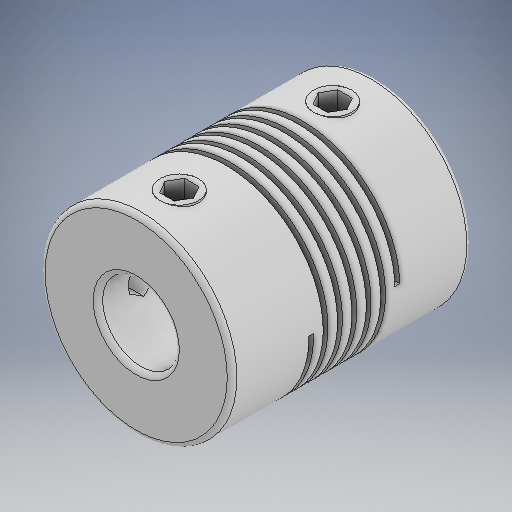
# Autodesk Inventor part: shaft_coupler 5mm_to_8mm
Saved by Autodesk Inventor 2025.2 (Build 292293000, 293)
## iProperties
Created: 2025-04-06
Part Number: shaft_coupler 5mm_to_8mm
Material: Generic
Document SubType Name: Modeling
Designer: Tiago
Density: 1 g/cm^3
Appearance: Default
Author: Tiago
Autodesk Inventor part; units mm, degrees
sketch "Sketch1" plane through (0, 0, 0) normal (0, 0, 1) x (1, 0, 0)
  circle A0 centre (0, 0) radius 10
  circle A1 centre (0, 0) radius 2.5
  dimension "D" = 20
  dimension "di1" = 5
  constraints: 2 centre point, 2 coincident
  measures "D" diameter of A0
  measures "di1" diameter of A1
ref_plane "Work Plane1" through (0, 0, 25) normal (0, 0, 1) x (1, 0, 0)
sketch "Sketch2" plane through (0, 0, 25) normal (0, 0, 1) x (1, 0, 0)
  circle A0 centre (0, 0) radius 4
  circle A1 centre (0, 0) radius 10
  dimension "di2" = 8
  dimension "d4" = 20
  constraints: 2 centre point, 2 coincident
  measures "di2" diameter of A0
  measures "d4" diameter of A1
extrude "Extrusion1" add sketch "Sketch2" against normal up to surface (25 mm away)
extrude "Extrusion2" add sketch "Sketch1" along normal blind 10
ref_plane "Work Plane2" through (-10, 0, 0) normal (1, 0, 0) x (0, 1, 0)
sketch "Sketch3" plane through (-10, 0, 0) normal (1, 0, 0) x (0, 1, 0)
  line L0 (0, 0) -> (0, 25) construction
  line L1 (-4, 25) -> (4, 25) construction
  line L2 (0, 20.5) -> (0, 4.5) construction
  circle A0 centre (0, 4.5) radius 2
  circle A1 centre (0, 4.5) radius 1.5 construction
  line L3 (1.5, 4.5) -> (0.75, 3.201)
  line L4 (0.75, 3.201) -> (-0.75, 3.201)
  line L5 (-0.75, 3.201) -> (-1.5, 4.5)
  line L6 (-1.5, 4.5) -> (-0.75, 5.799)
  line L7 (-0.75, 5.799) -> (0.75, 5.799)
  line L8 (0.75, 5.799) -> (1.5, 4.5)
  line L9 (0, 12.5) -> (3.6503, 12.5)
  line L10 (0, 25) -> (0, 0) construction
  line L11 (0, 4.5) -> (0, 20.5) construction
  circle A2 centre (0, 20.5) radius 2
  circle A3 centre (0, 20.5) radius 1.5 construction
  line L12 (1.5, 20.5) -> (0.75, 21.799)
  line L13 (0.75, 21.799) -> (-0.75, 21.799)
  line L14 (-0.75, 21.799) -> (-1.5, 20.5)
  line L15 (-1.5, 20.5) -> (-0.75, 19.201)
  line L16 (-0.75, 19.201) -> (0.75, 19.201)
  line L17 (0.75, 19.201) -> (1.5, 20.5)
  dimension "HH" = 3
  dimension "d14" = 16
  dimension "M" = 4
  constraints: 34 end point, 13 symmetric about line, 6 coincident, 3 midpoint, 2 centre point, 2 horizontal, 2 horizontal alignment, 2 point on line, 18 other
  measures "d14" distance of L2.start L2.end
  measures "M" diameter of A0
ref_plane "Work Plane3" through (0, 10, 0) normal (0, 1, 0) x (-1, 0, 0)
sketch "Sketch5" plane through (0, 10, 0) normal (0, 1, 0) x (-1, 0, 0)
  line L0 (0, 0) -> (0, 25) construction
  line L1 (0, 20.5) -> (0, 4.5) construction
  circle A0 centre (0, 4.5) radius 2
  circle A1 centre (0, 4.5) radius 1.5 construction
  line L2 (1.5, 4.5) -> (0.75, 3.201)
  line L3 (0.75, 3.201) -> (-0.75, 3.201)
  line L4 (-0.75, 3.201) -> (-1.5, 4.5)
  line L5 (-1.5, 4.5) -> (-0.75, 5.799)
  line L6 (-0.75, 5.799) -> (0.75, 5.799)
  line L7 (0.75, 5.799) -> (1.5, 4.5)
  line L8 (0, 12.5) -> (3.6503, 12.5)
  line L9 (0, 25) -> (0, 0) construction
  line L10 (0, 4.5) -> (0, 20.5) construction
  circle A2 centre (0, 20.5) radius 2
  circle A3 centre (0, 20.5) radius 1.5 construction
  line L11 (1.5, 20.5) -> (0.75, 21.799)
  line L12 (0.75, 21.799) -> (-0.75, 21.799)
  line L13 (-0.75, 21.799) -> (-1.5, 20.5)
  line L14 (-1.5, 20.5) -> (-0.75, 19.201)
  line L15 (-0.75, 19.201) -> (0.75, 19.201)
  line L16 (0.75, 19.201) -> (1.5, 20.5)
  dimension "d20" = 3
  dimension "d18" = 16
  dimension "d19" = 4
  constraints: 34 end point, 13 symmetric about line, 6 coincident, 2 centre point, 2 horizontal, 2 horizontal alignment, 2 midpoint, 2 point on line, 18 other
  measures "d18" distance of L1.start L1.end
  measures "d19" diameter of A0
fillet "Fillet1" radius 0.5 4 edges at (-10, 0, 0) (-10, 0, 25) (-2.5, 0, 0) (-4, 0, 25)
extrude "Extrusion3" cut sketch "Sketch3" along normal up to surface contours L3 L4 L5 L6 L7 L8 | L17 L16 L15 L14 L13 L12 round surface about axis through (0, 0, 0) along (0, 0, 1) radius 2.5 far side no
extrude "Extrusion4" add sketch "Sketch3" along normal up to surface round surface about axis through (0, 0, 25) along (0, 0, -1) radius 10 far side no
extrude "Extrusion5" cut sketch "Sketch5" against normal up to surface contours L2 L3 L4 L5 L6 L7 | L16 L15 L14 L13 L12 L11 round surface about axis through (0, 0, 0) along (0, 0, 1) radius 2.5 far side no
extrude "Extrusion6" add sketch "Sketch5" along normal up to surface round surface about axis through (0, 0, 25) along (0, 0, -1) radius 10 far side no
sketch "Sketch6" plane through (0, 0, 0) normal (0, 1, 0) x (-1, 0, 0)
  line L0 (10, 6.5) -> (10, 5.799) projected
  line L1 (10, 5.799) -> (2.5, 5.799) projected
  line L2 (2.5, 5.799) -> (2.5, 10) projected
  line L3 (2.5, 10) -> (4, 10) projected
  line L4 (4, 10) -> (4, 19.201) projected
  line L5 (4, 19.201) -> (10, 19.201) projected
  line L6 (10, 19.201) -> (10, 18.5) projected
  line L7 (10, 18.5) -> (10, 6.5) projected
  arc A0 (4.5, 25) -> (4, 24.5) centre (4.5, 24.5) ccw projected
  line L8 (4.5, 25) -> (9.5, 25) projected
  arc A1 (10, 24.5) -> (9.5, 25) centre (9.5, 24.5) ccw projected
  line L9 (10, 24.5) -> (10, 22.5) projected
  line L10 (10, 22.5) -> (10, 21.799) projected
  line L11 (10, 21.799) -> (4, 21.799) projected
  line L12 (4, 21.799) -> (4, 24.5) projected
  arc A2 (-3, 0) -> (-2.5, 0.5) centre (-3, 0.5) ccw projected
  line L13 (-3, 0) -> (-9.5, 0) projected
  arc A3 (-10, 0.5) -> (-9.5, 0) centre (-9.5, 0.5) ccw projected
  line L14 (-10, 0.5) -> (-10, 24.5) projected
  arc A4 (-9.5, 25) -> (-10, 24.5) centre (-9.5, 24.5) ccw projected
  line L15 (-9.5, 25) -> (-4.5, 25) projected
  arc A5 (-4, 24.5) -> (-4.5, 25) centre (-4.5, 24.5) ccw projected
  line L16 (-4, 24.5) -> (-4, 10) projected
  line L17 (-4, 10) -> (-2.5, 10) projected
  line L18 (-2.5, 10) -> (-2.5, 0.5) projected
  arc A6 (2.5, 0.5) -> (3, 0) centre (3, 0.5) ccw projected
  line L19 (2.5, 0.5) -> (2.5, 3.201) projected
  line L20 (2.5, 3.201) -> (10, 3.201) projected
  line L21 (10, 3.201) -> (10, 2.5) projected
  line L22 (10, 2.5) -> (10, 0.5) projected
  arc A7 (9.5, 0) -> (10, 0.5) centre (9.5, 0.5) ccw projected
  line L23 (9.5, 0) -> (3, 0) projected
  line L24 (-10, 0) -> (-10, 7.5) construction
  line L25 (-10, 25) -> (-10, 17.5) construction
  line L26 (-10, 7.5) -> (-10, 8.5)
  line L27 (-10, 7.5) -> (-6, 7.5)
  line L28 (-6, 7.5) -> (-6, 8)
  line L29 (-6, 8) -> (-10, 8)
  point P0 (0, 0)
  dimension "d30" = 7.5
  dimension "d31" = 7.5
  dimension "d32" = 1
  dimension "d33" = 4
  dimension "d34" = 0.5
  constraints: 12 end point, 3 point on line, 1 horizontal, 1 midpoint, 1 perpendicular
  measures "d30" distance of L24.start L24.end
  measures "d31" distance of L25.start L25.end
  measures "d32" distance of L24.end L26.end
  measures "d33" distance of L24.end L27.end
  measures "d34" distance of L27.end L28.end
coil "Coil1" sketch "Sketch6" operation cut axis through (0, 0, -10) along (0, 0, 1) pitch 1.5 turns 6 hand right contours L14 L29 L28 L27
equation "\"d4\" = D"
body "Solid2"
